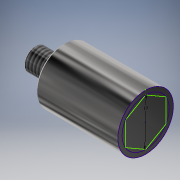
# Autodesk Inventor part: Albero cuscinetto
Saved by Autodesk Inventor 2018 (Build 220112000, 112)
## iProperties
Created: 2020-05-28
Part Number: Albero cuscinetto
Material: Generico
Document SubType Name: Modeling
Designer: Francesco
Density: 1 g/cm^3
Appearance: Acciaio - Lucido
Author: Francesco
Autodesk Inventor part; units mm, degrees
ref_plane "YZ Plane" through (0, 0, 0) normal (1, 0, 0) x (0, 1, 0)
ref_plane "XZ Plane" through (0, 0, 0) normal (0, 1, 0) x (-1, 0, 0)
ref_plane "XY Plane" through (0, 0, 0) normal (0, 0, 1) x (1, 0, 0)
sketch "Schizzo1" plane through (0, 0, 0) normal (0, 0, 1) x (1, 0, 0)
  line L0 (-25, 0) -> (42.5, 0)
  line L1 (-25, 0) -> (-25, 4)
  line L2 (-25, 4) -> (-15, 4)
  line L3 (-15, 4) -> (-15, 10)
  line L4 (-15, 10) -> (15, 10)
  line L5 (15, 10) -> (15, 0)
  point P0 (0, 0)
  point P1 (0, 0)
  point P2 (15, 4)
  point P3 (42.5, 4)
  point P4 (0, 10)
  dimension "d0" = 8
  dimension "d1" = 10
  dimension "d2" = 20
  dimension "d3" = 30
  constraints: 13 end point, 5 point on line, 4 perpendicular, 2 coincident, 1 horizontal, 1 midpoint, 1 vertical, 1 vertical alignment
  measures "d0" diameter of L2 L0
  measures "d1" distance between parallel lines of L3 L1
  measures "d2" diameter of L4 L0
  measures "d3" distance of L3.end L4.end
revolve "Rivoluzione1" add sketch "Schizzo1" angle 360 about axis through (-25, 0, 0) along (1, 0, 0)
chamfer "Smusso1" distance 0.5 angle 45 1 edges at (-25, -4, 0)
thread "Filettatura1" size "M8x1.25" class "6g" standard "ISO Metric profile" full length
chamfer "Smusso2" distance 1 angle 45 1 edges at (-15, -10, 0)
sketch "Schizzo2" plane through (15, 0, 0) normal (1, 0, 0) x (0, 0, -1)
  circle A0 centre (0, 0) radius 10 projected
  circle A1 centre (0, 0) radius 10
  line L0 (-8.5, 0) -> (-4.25, 7.3612)
  line L1 (-4.25, 7.3612) -> (4.25, 7.3612)
  line L2 (4.25, 7.3612) -> (8.5, 0)
  line L3 (8.5, 0) -> (4.25, -7.3612)
  line L4 (4.25, -7.3612) -> (-4.25, -7.3612)
  line L5 (-4.25, -7.3612) -> (-8.5, 0)
  point P0 (0, 0)
  point P1 (0, 0)
  point P2 (-10, 0)
  dimension "d17" = 17
  constraints: 12 end point, 2 coincident, 2 horizontal alignment, 16 other
  measures "d17" distance of L2.end L0.start
extrude "Estrusione2" cut sketch "Schizzo2" against normal blind 8
